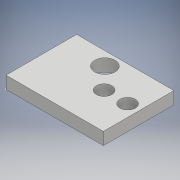
# Autodesk Inventor part: SensorPCB
Saved by Autodesk Inventor 2018 (Build 220112000, 112)
## iProperties
Created: 2018-05-09
Part Number: SensorPCB
Material: Generic
Document SubType Name: Modeling
Designer: s4321966
Density: 1 g/cm^3
Appearance: Default
Mass: 0.323283 g
Surface Area: 4.84166 cm^2
Volume: 0.323283 cm^3
Author: s4321966
Autodesk Inventor part; units mm, degrees
ref_plane "YZ Plane" through (0, 0, 0) normal (1, 0, 0) x (0, 1, 0)
ref_plane "XZ Plane" through (0, 0, 0) normal (0, 1, 0) x (-1, 0, 0)
ref_plane "XY Plane" through (0, 0, 0) normal (0, 0, 1) x (1, 0, 0)
sketch "Sketch1" plane through (0, 0, 0) normal (0, 0, 1) x (1, 0, 0)
  point P0 (0, 0)
sketch "Sketch2" plane through (0, 0, 0) normal (0, 0, 1) x (1, 0, 0)
  line L0 (0, 0) -> (15.75, 0)
  line L1 (15.75, 0) -> (15.75, 11.43)
  line L2 (15.75, 11.43) -> (0, 11.43)
  line L3 (0, 11.43) -> (0, 0)
  dimension "d0" = 15.75
  dimension "d1" = 11.43
  constraints: 8 end point, 2 parallel, 1 horizontal, 1 perpendicular
  measures "d0" distance of L2.end L1.end
  measures "d1" distance of L1.end L0.end
extrude "Extrusion1" add sketch "Sketch2" along normal blind 2
sketch "Sketch3" plane through (0, 0, 2) normal (0, 0, 1) x (1, 0, 0)
  line L0 (15.75, 11.43) -> (0, 11.43) projected
  line L1 (0, 11.43) -> (6.73, 11.43)
  line L2 (0, 11.43) -> (6.73, 11.43) construction
  line L3 (6.73, 11.43) -> (6.73, 9.27)
  circle A0 centre (6.73, 9.27) radius 1.651
  line L4 (15.75, 11.43) -> (13.84, 11.43)
  line L5 (15.75, 11.43) -> (17.66, 11.43) construction
  line L6 (13.84, 11.43) -> (13.84, 5.84)
  line L7 (13.84, 5.84) -> (10.04, 5.84)
  circle A1 centre (10.04, 5.84) radius 1.25
  circle A2 centre (13.84, 5.84) radius 1.25
  point P0 (0, 0)
  dimension "d4" = 6.73
  dimension "d5" = 0
  dimension "d6" = 2.16
  dimension "d7" = 90
  dimension "d8" = 3.302
  dimension "d9" = 1.91
  dimension "d10" = 180
  dimension "d11" = 5.59
  dimension "d12" = 90
  dimension "d13" = 3.8
  dimension "d14" = 90
  dimension "d15" = 2.5
  dimension "d16" = 2.5
  constraints: 14 end point, 3 centre point, 3 coincident, 3 collinear, 3 horizontal, 3 perpendicular
  measures "d4" distance of L0.end L1.end
  measures "d5" distance between parallel lines of L1 L2
  measures "d6" distance of L1.end L3.end
  measures "d7" angle of L1 L3
  measures "d8" diameter of A0
  measures "d9" distance of L0.start L4.end
  measures "d10" angle of L4 L5
  measures "d11" distance of L4.end L6.end
  measures "d12" angle of L6 L4
  measures "d13" distance of L6.end L7.end
  measures "d14" angle of L6 L7
  measures "d15" diameter of A1
  measures "d16" diameter of A2
extrude "Extrusion2" cut sketch "Sketch3" against normal blind 2
body "Solid1"
